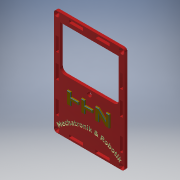
# Autodesk Inventor part: Deckplatte
Saved by Autodesk Inventor 2019 (Build 230136000, 136)
## iProperties
Created: 2022-10-31
Part Number: Deckplatte
Material: Generisch
Document SubType Name: Modeling
Designer: RP
Density: 1 g/cm^3
Appearance: Hellrot
Author: RP
Autodesk Inventor part; units mm, degrees
ref_plane "YZ Plane" through (0, 0, 0) normal (1, 0, 0) x (0, 1, 0)
ref_plane "XZ Plane" through (0, 0, 0) normal (0, 1, 0) x (-1, 0, 0)
sketch "Skizze1" plane through (0, 0, 0) normal (0, 0, 1) x (1, 0, 0)
  line L0 (92, 4) -> (0, 4)
  line L1 (96, -142) -> (96, 0)
  arc A0 (96, 0) -> (92, 4) centre (92, 0) ccw
  arc A1 (0, 4) -> (-4, 0) centre (0, 0) ccw
  line L2 (-4, 0) -> (-4, -142)
  arc A2 (-4, -142) -> (0, -146) centre (0, -142) ccw
  line L3 (0, -146) -> (92, -146)
  arc A3 (92, -146) -> (96, -142) centre (92, -142) ccw
  circle A4 centre (92, -142) radius 1.75
  circle A5 centre (0, -142) radius 1.75
  line L4 (37.25, -139.5) -> (17.25, -139.5)
  line L5 (17.25, -143.5) -> (37.25, -143.5)
  line L6 (17.25, -139.5) -> (17.25, -143.5)
  line L7 (37.25, -143.5) -> (37.25, -139.5)
  line L8 (54.75, -139.5) -> (54.75, -143.5)
  line L9 (74.75, -139.5) -> (54.75, -139.5)
  line L10 (54.75, -143.5) -> (74.75, -143.5)
  line L11 (74.75, -143.5) -> (74.75, -139.5)
  line L12 (89.5, -104.75) -> (89.5, -124.75)
  line L13 (93.5, -104.75) -> (89.5, -104.75)
  line L14 (93.5, -124.75) -> (93.5, -104.75)
  line L15 (89.5, -124.75) -> (93.5, -124.75)
  line L16 (93.5, -81) -> (93.5, -61)
  line L17 (89.5, -61) -> (89.5, -81)
  line L18 (89.5, -81) -> (93.5, -81)
  line L19 (93.5, -61) -> (89.5, -61)
  line L20 (89.5, -47) -> (93.5, -47)
  line L21 (93.5, -27) -> (89.5, -27)
  line L22 (93.5, -47) -> (93.5, -27)
  line L23 (89.5, -27) -> (89.5, -47)
  circle A6 centre (92, 0) radius 1.75
  line L24 (54.75, -2.5) -> (74.75, -2.5)
  line L25 (74.75, -2.5) -> (74.75, 1.5)
  line L26 (74.75, 1.5) -> (54.75, 1.5)
  line L27 (54.75, 1.5) -> (54.75, -2.5)
  line L28 (37.25, -2.5) -> (37.25, 1.5)
  line L29 (17.25, 1.5) -> (17.25, -2.5)
  line L30 (37.25, 1.5) -> (17.25, 1.5)
  line L31 (17.25, -2.5) -> (37.25, -2.5)
  circle A7 centre (0, 0) radius 1.75
  line L32 (2.5, -47) -> (2.5, -27)
  line L33 (-1.5, -27) -> (-1.5, -47)
  line L34 (2.5, -27) -> (-1.5, -27)
  line L35 (-1.5, -47) -> (2.5, -47)
  line L36 (2.5, -61) -> (-1.5, -61)
  line L37 (-1.5, -81) -> (2.5, -81)
  line L38 (2.5, -81) -> (2.5, -61)
  line L39 (-1.5, -61) -> (-1.5, -81)
  line L40 (-1.5, -104.75) -> (-1.5, -124.75)
  line L41 (2.5, -104.75) -> (-1.5, -104.75)
  line L42 (-1.5, -124.75) -> (2.5, -124.75)
  line L43 (2.5, -124.75) -> (2.5, -104.75)
  line L44 (4.4, -8) -> (87.6, -8)
  line L45 (87.6, -8) -> (87.6, -69.6)
  line L46 (87.6, -69.6) -> (4.4, -69.6)
  line L47 (4.4, -69.6) -> (4.4, -8)
  circle A8 centre (46, -76) radius 3.25
  line L48 (-4, -76) -> (96, -76) construction
  dimension "d0" = 8
  dimension "d1" = 4.4
  dimension "d2" = 4.4
  dimension "d3" = 69.6
  dimension "d7" = 6.5
  dimension "d8" = 76
  constraints: 98 end point, 23 horizontal, 22 vertical, 9 centre point, 8 point on circle, 2 parallel, 2 perpendicular, 2 point on line, 1 coincident, 1 midpoint, 64 other
  measures "d0" distance from line of L44 A0.centre
  measures "d1" distance from line of A0.centre L45
  measures "d2" distance from line of point (0, 0) L47
  measures "d3" distance from line of point (0, 0) L46
  measures "d7" diameter of A8
  measures "d8" vertical distance of point (0, 0) point (46, -76)
extrude "Extrusion1" add sketch "Skizze1" against normal blind 4
fillet "Rundung1" radius 6.6 2 edges at (4.4, -69.6, -2) (87.6, -69.6, -2)
chamfer "Fase2" distance 4 angle 45 1 edges at (46, -8, -4) measured on face at (46, -8, -3.5)
chamfer "Fase3" distance 2.2 angle 45 4 edges at (-1.75, -142, 0) (90.25, -142, 0) (-1.75, 0, 0) (90.25, 0, 0)
sketch "Skizze2" plane through (0, 0, 0) normal (0, 0, 1) x (1, 0, 0)
  line L0 (16, -85) -> (16, -102.0769)
  line L1 (16, -102.0769) -> (20.99, -102.0769)
  line L2 (20.99, -102.0769) -> (20.99, -95.5345)
  line L3 (20.99, -95.5345) -> (32.008, -95.5345)
  line L4 (32.008, -95.5345) -> (32.008, -91.5425)
  line L5 (32.008, -91.5425) -> (20.99, -91.5425)
  line L6 (20.99, -91.5425) -> (20.99, -85)
  line L7 (20.99, -85) -> (16, -85)
  line L8 (36, -85) -> (36, -102.0769)
  line L9 (36, -102.0769) -> (40.99, -102.0769)
  line L10 (40.99, -102.0769) -> (40.99, -95.5345)
  line L11 (40.99, -95.5345) -> (52.008, -95.5345)
  line L12 (52.008, -95.5345) -> (52.008, -91.5425)
  line L13 (52.008, -91.5425) -> (40.99, -91.5425)
  line L14 (40.99, -85) -> (40.99, -91.5425)
  line L15 (36, -85) -> (40.99, -85)
  line L16 (56, -85) -> (56, -102.0769)
  line L17 (56, -102.0769) -> (60.99, -102.0769)
  line L18 (71.01, -102.0769) -> (76, -102.0769)
  line L19 (76, -102.0769) -> (76, -85)
  line L20 (76, -85) -> (71.01, -85)
  line L21 (56, -85) -> (60.99, -85)
  circle A0 centre (92, 0) radius 1.75 construction
  circle A1 centre (92, -142) radius 1.75 construction
  circle A2 centre (0, -142) radius 1.75 construction
  line L22 (0, 0) -> (92, 0) construction
  line L23 (92, 0) -> (92, -142) construction
  line L24 (92, -142) -> (0, -142) construction
  line L25 (0, -142) -> (0, 0) construction
  line L26 (32.008, -93.5385) -> (16, -93.5385) construction
  line L27 (52.008, -93.5385) -> (36, -93.5385) construction
  line L28 (36, -93.5385) -> (32.008, -93.5385) construction
  line L29 (76, -93.5385) -> (56, -93.5385) construction
  line L30 (56, -93.5385) -> (52.008, -93.5385) construction
  line L31 (16, -85) -> (36, -85) construction
  line L32 (56, -85) -> (36, -85) construction
  line L33 (76, -85) -> (56, -85) construction
  line L34 (46, -76) -> (46, -60.5619) construction
  circle A3 centre (0, 0) radius 3.95 construction
  circle A4 centre (0, -142) radius 3.95 construction
  line L35 (4.4, -63) -> (4.4, -8) construction
  line L36 (87.6, -8) -> (87.6, -63) construction
  arc A5 (81, -69.6) -> (87.6, -63) centre (81, -63) ccw construction
  line L37 (81, -69.6) -> (11, -69.6) projected
  arc A6 (4.4, -63) -> (11, -69.6) centre (11, -63) ccw construction
  line L38 (2.5, -124.75) -> (-1.5, -124.75) construction
  line L39 (-1.5, -124.75) -> (-1.5, -104.75) construction
  line L40 (-1.5, -104.75) -> (2.5, -104.75) construction
  line L41 (2.5, -104.75) -> (2.5, -124.75) construction
  line L42 (-1.5, -81) -> (-1.5, -61) construction
  line L43 (-1.5, -61) -> (2.5, -61) construction
  line L44 (2.5, -61) -> (2.5, -81) construction
  line L45 (2.5, -81) -> (-1.5, -81) construction
  line L46 (-1.5, -27) -> (2.5, -27) construction
  line L47 (2.5, -27) -> (2.5, -47) construction
  line L48 (2.5, -47) -> (-1.5, -47) construction
  line L49 (-1.5, -47) -> (-1.5, -27) construction
  line L50 (17.25, 1.5) -> (37.25, 1.5) construction
  line L51 (37.25, 1.5) -> (37.25, -2.5) construction
  line L52 (37.25, -2.5) -> (17.25, -2.5) construction
  line L53 (17.25, -2.5) -> (17.25, 1.5) construction
  line L54 (74.75, 1.5) -> (74.75, -2.5) construction
  line L55 (74.75, -2.5) -> (54.75, -2.5) construction
  line L56 (54.75, -2.5) -> (54.75, 1.5) construction
  line L57 (54.75, 1.5) -> (74.75, 1.5) construction
  line L58 (93.5, -27) -> (93.5, -47) construction
  line L59 (93.5, -47) -> (89.5, -47) construction
  line L60 (89.5, -47) -> (89.5, -27) construction
  line L61 (89.5, -27) -> (93.5, -27) construction
  line L62 (89.5, -61) -> (93.5, -61) construction
  line L63 (93.5, -61) -> (93.5, -81) construction
  line L64 (93.5, -81) -> (89.5, -81) construction
  line L65 (89.5, -81) -> (89.5, -61) construction
  line L66 (93.5, -124.75) -> (89.5, -124.75) construction
  line L67 (89.5, -124.75) -> (89.5, -104.75) construction
  line L68 (89.5, -104.75) -> (93.5, -104.75) construction
  line L69 (93.5, -104.75) -> (93.5, -124.75) construction
  line L70 (74.75, -143.5) -> (54.75, -143.5) construction
  line L71 (54.75, -143.5) -> (54.75, -139.5) construction
  line L72 (54.75, -139.5) -> (74.75, -139.5) construction
  line L73 (74.75, -139.5) -> (74.75, -143.5) construction
  line L74 (17.25, -143.5) -> (17.25, -139.5) construction
  line L75 (17.25, -139.5) -> (37.25, -139.5) construction
  line L76 (37.25, -139.5) -> (37.25, -143.5) construction
  line L77 (37.25, -143.5) -> (17.25, -143.5) construction
  circle A7 centre (46, -76) radius 3.25 construction
  line L78 (92, 4) -> (0, 4) construction
  arc A8 (0, 4) -> (-4, 0) centre (0, 0) ccw construction
  line L79 (-4, 0) -> (-4, -142) construction
  arc A9 (-4, -142) -> (0, -146) centre (0, -142) ccw construction
  line L80 (0, -146) -> (92, -146) construction
  arc A10 (92, -146) -> (96, -142) centre (92, -142) ccw construction
  line L81 (96, -142) -> (96, 0) construction
  arc A11 (96, 0) -> (92, 4) centre (92, 0) ccw construction
  circle A12 centre (92, -142) radius 3.95 construction
  circle A13 centre (92, 0) radius 3.95 construction
  line L82 (71.01, -95.02) -> (60.99, -85)
  line L83 (71.01, -95.02) -> (71.01, -85)
  line L84 (60.99, -102.0769) -> (60.99, -92.0569)
  line L85 (60.99, -92.0569) -> (71.01, -102.0769)
  line L86 (73.2066, -97.2166) -> (69.6781, -100.7451) construction
  line L87 (4.4, -8) -> (87.6, -8) projected
  dimension "d19" = 60
  dimension "d20" = 45
  dimension "d22" = 3.992
  dimension "d23" = 4.99
  dimension "d24" = 17.0769
  dimension "d26" = 85
  dimension "d27" = 4.99
  constraints: 81 end point, 17 point on line, 16 perpendicular, 9 equal length, 6 midpoint, 5 collinear, 5 vertical, 3 horizontal, 3 parallel, 1 coincident, 1 other
  measures "d19" distance between parallel lines of L19 L0
  measures "d20" angle of L84 L85
  measures "d22" distance of L3.end L4.end
  measures "d23" distance between parallel lines of L2 L0
  measures "d24" distance between parallel lines of L1 L7
  measures "d26" distance from line of L7 L22.start
  measures "d27" distance between parallel lines of L82 L85
extrude "Extrusion2" add sketch "Skizze2" along normal blind 2
fillet "Rundung2" radius 0.5 25 edges at (26.499, -95.5345, 0) (20.99, -98.8057, 0) (18.495, -102.0769, 0) (32.008, -93.5385, 0) (40.99, -98.8057, 0) (46.499, -95.5345, 0) (38.495, -102.0769, 0) (58.495, -102.0769, 0) (60.99, -97.0669, 0) (66, -97.0669, 0) (73.505, -102.0769, 0) (76, -93.5385, 0) (73.505, -85, 0) (66, -90.01, 0) (58.495, -85, 0) (52.008, -93.5385, 0) (46.499, -91.5425, 0) (40.99, -88.2712, 0) (38.495, -85, 0) (26.499, -91.5425, 0) (20.99, -88.2712, 0) (18.495, -85, 0) (56, -93.5385, 0) (36, -93.5385, 0) (16, -93.5385, 0)
ref_plane "Arbeitsebene1" through (31.625, -139.5, 0) normal (0, -0.052336, 0.9986295) x (1, 0, 0)
sketch "Skizze3" plane through (31.625, -139.5, 0) normal (0, -0.052336, 0.9986295) x (1, 0, 0)
  arc A0 (52.375, 5.3883) -> (-23.625, 5.3883) centre (14.375, -43.5326) ccw construction
  ellipse E0 centre (14.375, 63.413) end of major axis (11.125, 63.413) minor radius 3.2455 construction
  line L0 (14.375, 63.413) -> (14.375, -10.3592) construction
  line L1 (14.375, -43.5326) -> (-23.625, 5.3883) construction
  line L2 (52.375, 5.3883) -> (14.375, -43.5326) construction
  ellipse E1 centre (-31.625, -2.6117) end of major axis (-33.375, -2.6117) minor radius 1.7476 construction
  line L3 (-35.625, 139.3088) -> (-35.625, -2.4966) construction
  line L4 (64.375, -2.4966) -> (64.375, 139.3088) construction
  line L5 (-23.8311, 5.3236) -> (-24.9638, 4.3439)
  line L6 (-24.9638, 4.3439) -> (-27.5657, 7.3521)
  line L7 (-27.5657, 7.3521) -> (-26.71, 4.6979)
  line L8 (-26.71, 4.6979) -> (-27.4896, 4.0236)
  line L9 (-27.4896, 4.0236) -> (-29.9928, 5.2529)
  line L10 (-29.9928, 5.2529) -> (-27.391, 2.2446)
  line L11 (-27.391, 2.2446) -> (-28.4648, 1.3159)
  line L12 (-28.4648, 1.3159) -> (-32.3899, 5.8539)
  line L13 (-32.3899, 5.8539) -> (-31.077, 6.9895)
  line L14 (-31.077, 6.9895) -> (-28.1323, 5.6214)
  line L15 (-28.1323, 5.6214) -> (-29.069, 8.7261)
  line L16 (-29.069, 8.7261) -> (-27.7562, 9.8617)
  line L17 (-27.7562, 9.8617) -> (-23.8311, 5.3236)
  spline S0 degree 2 poles (-20.9166, 7.2303) (-21.9657, 6.4907) (-23.7884, 6.7048) (-24.4412, 7.6307) knots 0 0 0 1 2 2 2
  spline S1 degree 2 poles (-24.4412, 7.6307) (-25.08, 8.5367) (-24.801, 10.3516) (-23.8632, 11.0129) knots 0 0 0 1 2 2 2
  spline S2 degree 2 poles (-23.8632, 11.0129) (-23.0168, 11.6097) (-21.5112, 11.2969) (-20.9116, 10.4465) knots 0 0 0 1 2 2 2
  line L18 (-20.9116, 10.4465) -> (-20.6174, 10.0293)
  line L19 (-20.6174, 10.0293) -> (-23.1487, 8.2445)
  spline S3 degree 2 poles (-23.1487, 8.2445) (-22.9507, 7.9974) (-22.523, 7.7873) (-22.2991, 7.7905) knots 0 0 0 1 2 2 2
  spline S4 degree 2 poles (-22.2991, 7.7905) (-22.0793, 7.7908) (-21.6202, 7.9836) (-21.3858, 8.1489) knots 0 0 0 1 2 2 2
  spline S5 degree 2 poles (-21.3858, 8.1489) (-21.1871, 8.289) (-20.8593, 8.651) (-20.7496, 8.8414) knots 0 0 0 1 2 2 2
  spline S6 degree 2 poles (-20.7496, 8.8414) (-20.6486, 9.0018) (-20.5138, 9.317) (-20.4775, 9.4259) knots 0 0 0 1 2 2 2
  line L20 (-20.4775, 9.4259) -> (-20.3544, 9.5127)
  line L21 (-20.3544, 9.5127) -> (-19.6819, 8.559)
  spline S7 degree 2 poles (-19.6819, 8.559) (-19.7857, 8.4025) (-19.949, 8.1446) (-20.122, 7.9512) knots 0 0 0 1 2 2 2
  spline S8 degree 2 poles (-20.122, 7.9512) (-20.2723, 7.7679) (-20.6305, 7.4321) (-20.9166, 7.2303) knots 0 0 0 1 2 2 2
  spline S9 degree 2 poles (-22.2442, 9.9233) (-22.51, 10.2833) (-23.1036, 10.4418) (-23.4334, 10.2093) knots 0 0 0 1 2 2 2
  spline S10 degree 2 poles (-23.4334, 10.2093) (-23.7712, 9.9711) (-23.8669, 9.2968) (-23.643, 8.9371) knots 0 0 0 1 2 2 2
  line L22 (-23.643, 8.9371) -> (-22.2442, 9.9233)
  spline S11 degree 2 poles (-16.8843, 9.8097) (-17.364, 9.5225) (-18.3057, 9.2874) (-18.7517, 9.3604) knots 0 0 0 1 2 2 2
  spline S12 degree 2 poles (-18.7517, 9.3604) (-19.1919, 9.4425) (-19.9744, 10.0111) (-20.2841, 10.5284) knots 0 0 0 1 2 2 2
  spline S13 degree 2 poles (-20.2841, 10.5284) (-20.6188, 11.0874) (-20.7354, 12.0773) (-20.5808, 12.51) knots 0 0 0 1 2 2 2
  spline S14 degree 2 poles (-20.5808, 12.51) (-20.4378, 12.9243) (-19.7934, 13.6274) (-19.3678, 13.8822) knots 0 0 0 1 2 2 2
  spline S15 degree 2 poles (-19.3678, 13.8822) (-19.0466, 14.0745) (-18.3143, 14.309) (-17.8915, 14.3411) knots 0 0 0 1 2 2 2
  line L23 (-17.8915, 14.3411) -> (-17.2721, 13.3065)
  line L24 (-17.2721, 13.3065) -> (-17.4264, 13.2141)
  spline S16 degree 2 poles (-17.4264, 13.2141) (-17.544, 13.24) (-17.8524, 13.282) (-18.0176, 13.2738) knots 0 0 0 1 2 2 2
  spline S17 degree 2 poles (-18.0176, 13.2738) (-18.196, 13.269) (-18.5855, 13.1718) (-18.7899, 13.0494) knots 0 0 0 1 2 2 2
  spline S18 degree 2 poles (-18.7899, 13.0494) (-19.253, 12.7722) (-19.3748, 11.8209) (-19.0451, 11.2702) knots 0 0 0 1 2 2 2
  spline S19 degree 2 poles (-19.0451, 11.2702) (-18.6955, 10.6862) (-17.8085, 10.4352) (-17.3579, 10.7049) knots 0 0 0 1 2 2 2
  spline S20 degree 2 poles (-17.3579, 10.7049) (-17.1285, 10.8423) (-16.8488, 11.1514) (-16.7686, 11.3014) knots 0 0 0 1 2 2 2
  spline S21 degree 2 poles (-16.7686, 11.3014) (-16.6901, 11.4447) (-16.6098, 11.7082) (-16.5847, 11.8082) knots 0 0 0 1 2 2 2
  line L25 (-16.5847, 11.8082) -> (-16.4303, 11.9006)
  line L26 (-16.4303, 11.9006) -> (-15.8084, 10.8619)
  spline S22 degree 2 poles (-15.8084, 10.8619) (-15.8853, 10.7535) (-16.0865, 10.4744) (-16.2058, 10.3519) knots 0 0 0 1 2 2 2
  spline S23 degree 2 poles (-16.2058, 10.3519) (-16.3511, 10.197) (-16.6298, 9.9621) (-16.8843, 9.8097) knots 0 0 0 1 2 2 2
  line L27 (-11.3125, 12.8763) -> (-12.5836, 12.2437)
  line L28 (-12.5836, 12.2437) -> (-13.5822, 14.2505)
  spline S24 degree 2 poles (-13.5822, 14.2505) (-13.7057, 14.4986) (-13.9875, 14.9666) (-14.096, 15.0538) knots 0 0 0 1 2 2 2
  spline S25 degree 2 poles (-14.096, 15.0538) (-14.2306, 15.1606) (-14.5329, 15.1569) (-14.7419, 15.0529) knots 0 0 0 1 2 2 2
  spline S26 degree 2 poles (-14.7419, 15.0529) (-14.8942, 14.9771) (-15.1535, 14.7014) (-15.2691, 14.4863) knots 0 0 0 1 2 2 2
  line L29 (-15.2691, 14.4863) -> (-13.8416, 11.6177)
  line L30 (-13.8416, 11.6177) -> (-15.1039, 10.9895)
  line L31 (-15.1039, 10.9895) -> (-17.8963, 16.6005)
  line L32 (-17.8963, 16.6005) -> (-16.6339, 17.2287)
  line L33 (-16.6339, 17.2287) -> (-15.6352, 15.222)
  spline S27 degree 2 poles (-15.6352, 15.222) (-15.4561, 15.637) (-15.0158, 16.2254) (-14.6589, 16.4031) knots 0 0 0 1 2 2 2
  spline S28 degree 2 poles (-14.6589, 16.4031) (-14.0407, 16.7107) (-12.9935, 16.2542) (-12.6252, 15.5142) knots 0 0 0 1 2 2 2
  line L34 (-12.6252, 15.5142) -> (-11.3125, 12.8763)
  spline S29 degree 2 poles (-8.2168, 14.6658) (-8.3073, 14.4989) (-8.4475, 14.2336) (-8.5922, 14.0712) knots 0 0 0 1 2 2 2
  spline S30 degree 2 poles (-8.5922, 14.0712) (-8.7341, 13.9152) (-9.0323, 13.6916) (-9.3304, 13.5728) knots 0 0 0 1 2 2 2
  spline S31 degree 2 poles (-9.3304, 13.5728) (-9.8905, 13.3495) (-10.9256, 13.8058) (-11.1524, 14.3749) knots 0 0 0 1 2 2 2
  spline S32 degree 2 poles (-11.1524, 14.3749) (-11.3379, 14.8401) (-11.1935, 15.5677) (-10.9078, 15.8753) knots 0 0 0 1 2 2 2
  spline S33 degree 2 poles (-10.9078, 15.8753) (-10.6194, 16.1891) (-9.6842, 16.7189) (-9.1296, 16.9819) knots 0 0 0 1 2 2 2
  line L35 (-9.1296, 16.9819) -> (-9.1386, 17.0045)
  spline S34 degree 2 poles (-9.1386, 17.0045) (-9.2772, 17.3523) (-9.8983, 17.4135) (-10.4132, 17.2082) knots 0 0 0 1 2 2 2
  spline S35 degree 2 poles (-10.4132, 17.2082) (-10.6435, 17.1164) (-11.2002, 16.7009) (-11.4416, 16.4528) knots 0 0 0 1 2 2 2
  line L36 (-11.4416, 16.4528) -> (-11.5545, 16.4078)
  line L37 (-11.5545, 16.4078) -> (-11.9596, 17.4241)
  spline S36 degree 2 poles (-11.9596, 17.4241) (-11.787, 17.5557) (-10.981, 18.0549) (-10.5384, 18.2314) knots 0 0 0 1 2 2 2
  spline S37 degree 2 poles (-10.5384, 18.2314) (-9.4544, 18.6635) (-8.1727, 18.3369) (-7.8774, 17.5962) knots 0 0 0 1 2 2 2
  line L38 (-7.8774, 17.5962) -> (-6.7377, 14.7372)
  line L39 (-6.7377, 14.7372) -> (-8.0385, 14.2186)
  line L40 (-8.0385, 14.2186) -> (-8.2168, 14.6658)
  line L41 (-8.476, 15.3162) -> (-8.8235, 16.1879)
  spline S38 degree 2 poles (-8.8235, 16.1879) (-9.1451, 16.023) (-9.5364, 15.8095) (-9.7063, 15.658) knots 0 0 0 1 2 2 2
  spline S39 degree 2 poles (-9.7063, 15.658) (-9.859, 15.5291) (-9.9515, 15.2096) (-9.8723, 15.0109) knots 0 0 0 1 2 2 2
  spline S40 degree 2 poles (-9.8723, 15.0109) (-9.7552, 14.7173) (-9.3463, 14.6238) (-9.0347, 14.748) knots 0 0 0 1 2 2 2
  spline S41 degree 2 poles (-9.0347, 14.748) (-8.8631, 14.8164) (-8.5648, 15.1185) (-8.476, 15.3162) knots 0 0 0 1 2 2 2
  spline S42 degree 2 poles (-4.0715, 15.5136) (-4.8906, 15.2496) (-5.8581, 15.6836) (-6.1057, 16.4518) knots 0 0 0 1 2 2 2
  line L42 (-6.1057, 16.4518) -> (-6.7545, 18.4649)
  line L43 (-6.7545, 18.4649) -> (-7.2682, 18.2994)
  line L44 (-7.2682, 18.2994) -> (-7.5695, 19.2342)
  line L45 (-7.5695, 19.2342) -> (-7.0558, 19.3997)
  line L46 (-7.0558, 19.3997) -> (-7.4526, 20.6307)
  line L47 (-7.4526, 20.6307) -> (-6.1106, 21.0633)
  line L48 (-6.1106, 21.0633) -> (-5.7138, 19.8323)
  line L49 (-5.7138, 19.8323) -> (-4.418, 20.25)
  line L50 (-4.418, 20.25) -> (-4.1167, 19.3151)
  line L51 (-4.1167, 19.3151) -> (-5.4125, 18.8975)
  line L52 (-5.4125, 18.8975) -> (-4.9188, 17.3657)
  spline S43 degree 2 poles (-4.9188, 17.3657) (-4.8457, 17.1389) (-4.7275, 16.8041) (-4.6287, 16.6878) knots 0 0 0 1 2 2 2
  spline S44 degree 2 poles (-4.6287, 16.6878) (-4.53, 16.5715) (-4.2062, 16.5021) (-3.947, 16.5857) knots 0 0 0 1 2 2 2
  spline S45 degree 2 poles (-3.947, 16.5857) (-3.836, 16.6215) (-3.5187, 16.8259) (-3.4612, 16.8853) knots 0 0 0 1 2 2 2
  line L53 (-3.4612, 16.8853) -> (-3.3455, 16.9226)
  line L54 (-3.3455, 16.9226) -> (-3.0413, 15.9785)
  spline S46 degree 2 poles (-3.0413, 15.9785) (-3.2409, 15.8529) (-3.7105, 15.63) (-4.0715, 15.5136) knots 0 0 0 1 2 2 2
  line L55 (-0.3403, 19.9438) -> (-0.4532, 19.9144)
  spline S47 degree 2 poles (-0.4532, 19.9144) (-0.5405, 19.9217) (-0.8443, 19.8726) (-1.0231, 19.826) knots 0 0 0 1 2 2 2
  spline S48 degree 2 poles (-1.0231, 19.826) (-1.2348, 19.7707) (-1.6768, 19.5197) (-1.8758, 19.3773) knots 0 0 0 1 2 2 2
  line L56 (-1.8758, 19.3773) -> (-1.1109, 16.4463)
  line L57 (-1.1109, 16.4463) -> (-2.4753, 16.0902)
  line L58 (-2.4753, 16.0902) -> (-3.6183, 20.4703)
  line L59 (-3.6183, 20.4703) -> (-2.2539, 20.8263)
  line L60 (-2.2539, 20.8263) -> (-2.0894, 20.1959)
  spline S49 degree 2 poles (-2.0894, 20.1959) (-2.0174, 20.3051) (-1.7569, 20.6545) (-1.6413, 20.7701) knots 0 0 0 1 2 2 2
  spline S50 degree 2 poles (-1.6413, 20.7701) (-1.5141, 20.8988) (-1.152, 21.129) (-0.978, 21.1744) knots 0 0 0 1 2 2 2
  spline S51 degree 2 poles (-0.978, 21.1744) (-0.9121, 21.1916) (-0.745, 21.2251) (-0.6779, 21.2376) knots 0 0 0 1 2 2 2
  line L61 (-0.6779, 21.2376) -> (-0.3403, 19.9438)
  spline S52 degree 2 poles (4.8407, 20.005) (5.0467, 18.9059) (4.0837, 17.4193) (2.9894, 17.2142) knots 0 0 0 1 2 2 2
  spline S53 degree 2 poles (2.9894, 17.2142) (1.8997, 17.0099) (0.4541, 18.0449) (0.2481, 19.1441) knots 0 0 0 1 2 2 2
  spline S54 degree 2 poles (0.2481, 19.1441) (0.0402, 20.2528) (1.0137, 21.7363) (2.1033, 21.9406) knots 0 0 0 1 2 2 2
  spline S55 degree 2 poles (2.1033, 21.9406) (3.1929, 22.1449) (4.6337, 21.109) (4.8407, 20.005) knots 0 0 0 1 2 2 2
  spline S56 degree 2 poles (3.4231, 19.7294) (3.3488, 20.1261) (3.1203, 20.6323) (2.976, 20.7685) knots 0 0 0 1 2 2 2
  spline S57 degree 2 poles (2.976, 20.7685) (2.8204, 20.9125) (2.4856, 20.9833) (2.2897, 20.9466) knots 0 0 0 1 2 2 2
  spline S58 degree 2 poles (2.2897, 20.9466) (2.0985, 20.9107) (1.8189, 20.7396) (1.7251, 20.5538) knots 0 0 0 1 2 2 2
  spline S59 degree 2 poles (1.7251, 20.5538) (1.6343, 20.3785) (1.5922, 19.8116) (1.6692, 19.4006) knots 0 0 0 1 2 2 2
  spline S60 degree 2 poles (1.6692, 19.4006) (1.7454, 18.9944) (1.9733, 18.5177) (2.1119, 18.3854) knots 0 0 0 1 2 2 2
  spline S61 degree 2 poles (2.1119, 18.3854) (2.2504, 18.253) (2.6118, 18.1724) (2.8126, 18.21) knots 0 0 0 1 2 2 2
  spline S62 degree 2 poles (2.8126, 18.21) (2.9798, 18.2414) (3.297, 18.4492) (3.3753, 18.6123) knots 0 0 0 1 2 2 2
  spline S63 degree 2 poles (3.3753, 18.6123) (3.4634, 18.802) (3.502, 19.3088) (3.4231, 19.7294) knots 0 0 0 1 2 2 2
  line L62 (10.2123, 18.3098) -> (8.7998, 18.1657)
  line L63 (8.7998, 18.1657) -> (8.5724, 20.3956)
  spline S64 degree 2 poles (8.5724, 20.3956) (8.5442, 20.6714) (8.4455, 21.2087) (8.3746, 21.3285) knots 0 0 0 1 2 2 2
  spline S65 degree 2 poles (8.3746, 21.3285) (8.2862, 21.4759) (8.002, 21.5789) (7.7698, 21.5552) knots 0 0 0 1 2 2 2
  spline S66 degree 2 poles (7.7698, 21.5552) (7.6005, 21.5379) (7.2608, 21.3713) (7.0767, 21.2108) knots 0 0 0 1 2 2 2
  line L64 (7.0767, 21.2108) -> (7.4019, 18.0231)
  line L65 (7.4019, 18.0231) -> (5.9991, 17.88)
  line L66 (5.9991, 17.88) -> (5.5398, 22.3834)
  line L67 (5.5398, 22.3834) -> (6.9425, 22.5265)
  line L68 (6.9425, 22.5265) -> (6.9934, 22.0283)
  spline S67 degree 2 poles (6.9934, 22.0283) (7.3072, 22.3535) (7.9266, 22.7491) (8.3233, 22.7895) knots 0 0 0 1 2 2 2
  spline S68 degree 2 poles (8.3233, 22.7895) (9.0102, 22.8596) (9.8294, 22.0634) (9.9133, 21.2411) knots 0 0 0 1 2 2 2
  line L69 (9.9133, 21.2411) -> (10.2123, 18.3098)
  line L70 (12.6662, 18.3934) -> (11.2572, 18.3385)
  line L71 (11.2572, 18.3385) -> (11.0809, 22.8618)
  line L72 (11.0809, 22.8618) -> (12.4898, 22.9167)
  line L73 (12.4898, 22.9167) -> (12.6662, 18.3934)
  line L74 (12.5084, 23.5646) -> (11.0168, 23.5065)
  line L75 (11.0168, 23.5065) -> (10.974, 24.6045)
  line L76 (10.974, 24.6045) -> (12.4656, 24.6626)
  line L77 (12.4656, 24.6626) -> (12.5084, 23.5646)
  line L78 (18.275, 18.3441) -> (16.5979, 18.3797)
  line L79 (16.5979, 18.3797) -> (15.4146, 20.3697)
  line L80 (15.4146, 20.3697) -> (15.1897, 20.0826)
  line L81 (15.1897, 20.0826) -> (15.1541, 18.4104)
  line L82 (15.1541, 18.4104) -> (13.7444, 18.4404)
  line L83 (13.7444, 18.4404) -> (13.8776, 24.7064)
  line L84 (13.8776, 24.7064) -> (15.2873, 24.6764)
  line L85 (15.2873, 24.6764) -> (15.2127, 21.1667)
  line L86 (15.2127, 21.1667) -> (16.5871, 22.9077)
  line L87 (16.5871, 22.9077) -> (18.2545, 22.8723)
  line L88 (18.2545, 22.8723) -> (16.6283, 20.9566)
  line L89 (16.6283, 20.9566) -> (18.275, 18.3441)
  line L90 (27.1946, 17.1705) -> (25.4212, 17.4428)
  line L91 (25.4212, 17.4428) -> (24.9789, 18.0223)
  spline S69 degree 2 poles (24.9789, 18.0223) (24.5091, 17.7501) (23.5902, 17.5961) (23.1096, 17.6699) knots 0 0 0 1 2 2 2
  spline S70 degree 2 poles (23.1096, 17.6699) (22.0859, 17.8271) (21.0642, 19.022) (21.1897, 19.839) knots 0 0 0 1 2 2 2
  spline S71 degree 2 poles (21.1897, 19.839) (21.2435, 20.1898) (21.5063, 20.6512) (21.6862, 20.8302) knots 0 0 0 1 2 2 2
  spline S72 degree 2 poles (21.6862, 20.8302) (21.8544, 20.9962) (22.2776, 21.2215) (22.4757, 21.2943) knots 0 0 0 1 2 2 2
  spline S73 degree 2 poles (22.4757, 21.2943) (22.3241, 21.4603) (22.0941, 21.7563) (22.0183, 21.9352) knots 0 0 0 1 2 2 2
  spline S74 degree 2 poles (22.0183, 21.9352) (21.9362, 22.1052) (21.881, 22.4827) (21.9186, 22.7278) knots 0 0 0 1 2 2 2
  spline S75 degree 2 poles (21.9186, 22.7278) (21.9585, 22.9873) (22.2411, 23.4505) (22.5139, 23.6251) knots 0 0 0 1 2 2 2
  spline S76 degree 2 poles (22.5139, 23.6251) (22.7645, 23.7834) (23.6021, 23.9204) (24.1308, 23.8392) knots 0 0 0 1 2 2 2
  spline S77 degree 2 poles (24.1308, 23.8392) (24.6066, 23.7662) (25.2683, 23.4628) (25.478, 23.2585) knots 0 0 0 1 2 2 2
  spline S78 degree 2 poles (25.478, 23.2585) (25.6781, 23.0556) (25.8501, 22.5421) (25.808, 22.2682) knots 0 0 0 1 2 2 2
  spline S79 degree 2 poles (25.808, 22.2682) (25.7815, 22.0952) (25.6071, 21.6645) (25.4493, 21.5018) knots 0 0 0 1 2 2 2
  spline S80 degree 2 poles (25.4493, 21.5018) (25.2623, 21.3091) (24.7093, 21.0399) (24.3049, 20.9692) knots 0 0 0 1 2 2 2
  line L92 (24.3049, 20.9692) -> (25.2749, 19.6937)
  line L93 (25.2749, 19.6937) -> (25.4768, 20.9761)
  line L94 (25.4768, 20.9761) -> (26.8657, 20.7628)
  line L95 (26.8657, 20.7628) -> (26.7978, 20.3207)
  spline S81 degree 2 poles (26.7978, 20.3207) (26.7727, 20.1573) (26.6316, 19.687) (26.5474, 19.5229) knots 0 0 0 1 2 2 2
  spline S82 degree 2 poles (26.5474, 19.5229) (26.4602, 19.3395) (26.1852, 18.9587) (25.9931, 18.7963) knots 0 0 0 1 2 2 2
  line L96 (25.9931, 18.7963) -> (27.2071, 17.2522)
  line L97 (27.2071, 17.2522) -> (27.1946, 17.1705)
  line L98 (24.4294, 18.8003) -> (23.0655, 20.5544)
  spline S83 degree 2 poles (23.0655, 20.5544) (22.989, 20.4727) (22.7655, 20.0741) (22.7301, 19.8435) knots 0 0 0 1 2 2 2
  spline S84 degree 2 poles (22.7301, 19.8435) (22.6895, 19.5791) (22.8083, 19.1673) (22.9325, 19.0154) knots 0 0 0 1 2 2 2
  spline S85 degree 2 poles (22.9325, 19.0154) (23.0575, 18.8684) (23.3932, 18.684) (23.571, 18.6567) knots 0 0 0 1 2 2 2
  spline S86 degree 2 poles (23.571, 18.6567) (23.8209, 18.6183) (24.2183, 18.6753) (24.4294, 18.8003) knots 0 0 0 1 2 2 2
  spline S87 degree 2 poles (24.3486, 22.3103) (24.3796, 22.5122) (24.3115, 22.7735) (24.2353, 22.8541) knots 0 0 0 1 2 2 2
  spline S88 degree 2 poles (24.2353, 22.8541) (24.168, 22.9284) (23.9905, 22.99) (23.9377, 22.9982) knots 0 0 0 1 2 2 2
  spline S89 degree 2 poles (23.9377, 22.9982) (23.88, 23.007) (23.7307, 22.9955) (23.6242, 22.943) knots 0 0 0 1 2 2 2
  spline S90 degree 2 poles (23.6242, 22.943) (23.5447, 22.906) (23.3973, 22.6827) (23.3722, 22.5193) knots 0 0 0 1 2 2 2
  spline S91 degree 2 poles (23.3722, 22.5193) (23.336, 22.2838) (23.5905, 21.8266) (23.8338, 21.5531) knots 0 0 0 1 2 2 2
  spline S92 degree 2 poles (23.8338, 21.5531) (24.0526, 21.6966) (24.3109, 22.0652) (24.3486, 22.3103) knots 0 0 0 1 2 2 2
  line L99 (35.225, 14.8847) -> (33.4693, 15.4118)
  line L100 (33.4693, 15.4118) -> (32.5054, 18.001)
  line L101 (32.5054, 18.001) -> (31.9839, 18.1576)
  line L102 (31.9839, 18.1576) -> (31.3505, 16.048)
  line L103 (31.3505, 16.048) -> (29.9162, 16.4787)
  line L104 (29.9162, 16.4787) -> (31.6416, 22.2253)
  line L105 (31.6416, 22.2253) -> (33.9514, 21.5317)
  spline S93 degree 2 poles (33.9514, 21.5317) (34.431, 21.3877) (35.1025, 21.0541) (35.3493, 20.7769) knots 0 0 0 1 2 2 2
  spline S94 degree 2 poles (35.3493, 20.7769) (35.5979, 20.4891) (35.778, 19.77) (35.6382, 19.3043) knots 0 0 0 1 2 2 2
  spline S95 degree 2 poles (35.6382, 19.3043) (35.441, 18.6477) (34.5974, 18.0024) (34.0265, 17.9098) knots 0 0 0 1 2 2 2
  line L106 (34.0265, 17.9098) -> (35.225, 14.8847)
  spline S96 degree 2 poles (34.1027, 19.5673) (34.1685, 19.7862) (34.0945, 20.1485) (33.9287, 20.2897) knots 0 0 0 1 2 2 2
  spline S97 degree 2 poles (33.9287, 20.2897) (33.8105, 20.3861) (33.4896, 20.518) (33.2428, 20.5921) knots 0 0 0 1 2 2 2
  line L107 (33.2428, 20.5921) -> (32.7585, 20.7375)
  line L108 (32.7585, 20.7375) -> (32.2943, 19.1914)
  line L109 (32.2943, 19.1914) -> (32.7087, 19.067)
  spline S98 degree 2 poles (32.7087, 19.067) (33.0068, 18.9775) (33.4529, 18.9248) (33.6322, 18.9978) knots 0 0 0 1 2 2 2
  spline S99 degree 2 poles (33.6322, 18.9978) (33.8055, 19.0677) (34.03, 19.3251) (34.1027, 19.5673) knots 0 0 0 1 2 2 2
  spline S100 degree 2 poles (40.423, 15.1993) (40.0071, 14.1612) (38.3968, 13.4235) (37.3632, 13.8377) knots 0 0 0 1 2 2 2
  spline S101 degree 2 poles (37.3632, 13.8377) (36.3342, 14.25) (35.6697, 15.899) (36.0856, 16.9371) knots 0 0 0 1 2 2 2
  spline S102 degree 2 poles (36.0856, 16.9371) (36.5051, 17.9842) (38.1226, 18.7138) (39.1517, 18.3015) knots 0 0 0 1 2 2 2
  spline S103 degree 2 poles (39.1517, 18.3015) (40.1807, 17.8892) (40.8407, 16.2419) (40.423, 15.1993) knots 0 0 0 1 2 2 2
  spline S104 degree 2 poles (39.0789, 15.7273) (39.229, 16.102) (39.3078, 16.6518) (39.2592, 16.8441) knots 0 0 0 1 2 2 2
  spline S105 degree 2 poles (39.2592, 16.8441) (39.2051, 17.0491) (38.9606, 17.2885) (38.7755, 17.3627) knots 0 0 0 1 2 2 2
  spline S106 degree 2 poles (38.7755, 17.3627) (38.595, 17.435) (38.2673, 17.4406) (38.0884, 17.3342) knots 0 0 0 1 2 2 2
  spline S107 degree 2 poles (38.0884, 17.3342) (37.9177, 17.2349) (37.578, 16.7792) (37.4225, 16.391) knots 0 0 0 1 2 2 2
  spline S108 degree 2 poles (37.4225, 16.391) (37.2687, 16.0074) (37.2053, 15.4828) (37.2512, 15.2968) knots 0 0 0 1 2 2 2
  spline S109 degree 2 poles (37.2512, 15.2968) (37.2971, 15.1108) (37.5588, 14.8488) (37.7484, 14.7728) knots 0 0 0 1 2 2 2
  spline S110 degree 2 poles (37.7484, 14.7728) (37.9064, 14.7095) (38.2856, 14.7147) (38.4391, 14.8104) knots 0 0 0 1 2 2 2
  spline S111 degree 2 poles (38.4391, 14.8104) (38.6153, 14.9231) (38.9198, 15.3302) (39.0789, 15.7273) knots 0 0 0 1 2 2 2
  spline S112 degree 2 poles (45.2655, 12.8764) (44.7823, 11.9112) (43.2076, 11.2097) (42.4815, 11.5733) knots 0 0 0 1 2 2 2
  spline S113 degree 2 poles (42.4815, 11.5733) (42.1815, 11.7235) (41.8012, 12.0825) (41.6208, 12.3522) knots 0 0 0 1 2 2 2
  line L110 (41.6208, 12.3522) -> (41.4685, 12.1783)
  line L111 (41.4685, 12.1783) -> (40.2598, 12.7835)
  line L112 (40.2598, 12.7835) -> (43.0657, 18.3877)
  line L113 (43.0657, 18.3877) -> (44.3266, 17.7564)
  line L114 (44.3266, 17.7564) -> (43.334, 15.7739)
  spline S114 degree 2 poles (43.334, 15.7739) (43.7319, 15.8737) (44.4539, 15.882) (44.8321, 15.6926) knots 0 0 0 1 2 2 2
  spline S115 degree 2 poles (44.8321, 15.6926) (45.5408, 15.3378) (45.7553, 13.8547) (45.2655, 12.8764) knots 0 0 0 1 2 2 2
  spline S116 degree 2 poles (43.9612, 13.4969) (44.2637, 14.1012) (44.1576, 14.8014) (43.775, 14.993) knots 0 0 0 1 2 2 2
  spline S117 degree 2 poles (43.775, 14.993) (43.6054, 15.0779) (43.2162, 15.1368) (43.0009, 15.1087) knots 0 0 0 1 2 2 2
  line L115 (43.0009, 15.1087) -> (41.9865, 13.0826)
  spline S118 degree 2 poles (41.9865, 13.0826) (42.0865, 12.9673) (42.3256, 12.8041) (42.4517, 12.741) knots 0 0 0 1 2 2 2
  spline S119 degree 2 poles (42.4517, 12.741) (42.9082, 12.5124) (43.6586, 12.8925) (43.9612, 13.4969) knots 0 0 0 1 2 2 2
  spline S120 degree 2 poles (49.782, 10.0797) (49.2, 9.1247) (47.4899, 8.6637) (46.5391, 9.2431) knots 0 0 0 1 2 2 2
  spline S121 degree 2 poles (46.5391, 9.2431) (45.5924, 9.82) (45.2099, 11.5563) (45.7919, 12.5112) knots 0 0 0 1 2 2 2
  spline S122 degree 2 poles (45.7919, 12.5112) (46.3789, 13.4745) (48.0948, 13.9264) (49.0415, 13.3495) knots 0 0 0 1 2 2 2
  spline S123 degree 2 poles (49.0415, 13.3495) (49.9881, 12.7726) (50.3665, 11.0388) (49.782, 10.0797) knots 0 0 0 1 2 2 2
  spline S124 degree 2 poles (48.5438, 10.8229) (48.7538, 11.1675) (48.9225, 11.6967) (48.9064, 11.8944) knots 0 0 0 1 2 2 2
  spline S125 degree 2 poles (48.9064, 11.8944) (48.887, 12.1055) (48.6854, 12.3821) (48.5152, 12.4858) knots 0 0 0 1 2 2 2
  spline S126 degree 2 poles (48.5152, 12.4858) (48.3491, 12.587) (48.0268, 12.6468) (47.8328, 12.5714) knots 0 0 0 1 2 2 2
  spline S127 degree 2 poles (47.8328, 12.5714) (47.6481, 12.5018) (47.2376, 12.1085) (47.02, 11.7515) knots 0 0 0 1 2 2 2
  spline S128 degree 2 poles (47.02, 11.7515) (46.8049, 11.3985) (46.6555, 10.8917) (46.67, 10.7007) knots 0 0 0 1 2 2 2
  spline S129 degree 2 poles (46.67, 10.7007) (46.6846, 10.5096) (46.8993, 10.2079) (47.0737, 10.1017) knots 0 0 0 1 2 2 2
  spline S130 degree 2 poles (47.0737, 10.1017) (47.219, 10.0131) (47.5939, 9.9555) (47.7611, 10.0244) knots 0 0 0 1 2 2 2
  spline S131 degree 2 poles (47.7611, 10.0244) (47.9535, 10.1065) (48.3211, 10.4575) (48.5438, 10.8229) knots 0 0 0 1 2 2 2
  spline S132 degree 2 poles (50.5708, 6.633) (49.8684, 7.1303) (49.6357, 8.1648) (50.102, 8.8236) knots 0 0 0 1 2 2 2
  line L116 (50.102, 8.8236) -> (51.3241, 10.5498)
  line L117 (51.3241, 10.5498) -> (50.8836, 10.8617)
  line L118 (50.8836, 10.8617) -> (51.4511, 11.6633)
  line L119 (51.4511, 11.6633) -> (51.8916, 11.3515)
  line L120 (51.8916, 11.3515) -> (52.6389, 12.4071)
  line L121 (52.6389, 12.4071) -> (53.7898, 11.5924)
  line L122 (53.7898, 11.5924) -> (53.0425, 10.5368)
  line L123 (53.0425, 10.5368) -> (54.1537, 9.7501)
  line L124 (54.1537, 9.7501) -> (53.5862, 8.9485)
  line L125 (53.5862, 8.9485) -> (52.475, 9.7351)
  line L126 (52.475, 9.7351) -> (51.5451, 8.4216)
  spline S133 degree 2 poles (51.5451, 8.4216) (51.4074, 8.2271) (51.2103, 7.9318) (51.1764, 7.783) knots 0 0 0 1 2 2 2
  spline S134 degree 2 poles (51.1764, 7.783) (51.1426, 7.6342) (51.2812, 7.3335) (51.5034, 7.1762) knots 0 0 0 1 2 2 2
  spline S135 degree 2 poles (51.5034, 7.1762) (51.5987, 7.1088) (51.9525, 6.9774) (52.0345, 6.967) knots 0 0 0 1 2 2 2
  line L127 (52.0345, 6.967) -> (52.1337, 6.8968)
  line L128 (52.1337, 6.8968) -> (51.5606, 6.0872)
  spline S136 degree 2 poles (51.5606, 6.0872) (51.3404, 6.1717) (50.8804, 6.4139) (50.5708, 6.633) knots 0 0 0 1 2 2 2
  line L129 (53.0949, 4.8256) -> (51.9843, 5.6943)
  line L130 (51.9843, 5.6943) -> (54.7732, 9.2599)
  line L131 (54.7732, 9.2599) -> (55.8839, 8.3912)
  line L132 (55.8839, 8.3912) -> (53.0949, 4.8256)
  line L133 (56.3167, 8.8736) -> (55.141, 9.7933)
  line L134 (55.141, 9.7933) -> (55.818, 10.6588)
  line L135 (55.818, 10.6588) -> (56.9937, 9.7391)
  line L136 (56.9937, 9.7391) -> (56.3167, 8.8736)
  line L137 (57.3429, 1.1629) -> (56.0862, 2.2741)
  line L138 (56.0862, 2.2741) -> (56.4694, 4.5573)
  line L139 (56.4694, 4.5573) -> (56.1123, 4.4837)
  line L140 (56.1123, 4.4837) -> (55.0044, 3.2306)
  line L141 (55.0044, 3.2306) -> (53.948, 4.1646)
  line L142 (53.948, 4.1646) -> (58.0995, 8.8599)
  line L143 (58.0995, 8.8599) -> (59.1558, 7.9259)
  line L144 (59.1558, 7.9259) -> (56.8305, 5.296)
  line L145 (56.8305, 5.296) -> (59.0045, 5.7362)
  line L146 (59.0045, 5.7362) -> (60.2539, 4.6315)
  line L147 (60.2539, 4.6315) -> (57.775, 4.2207)
  line L148 (57.775, 4.2207) -> (57.3429, 1.1629)
  point P0 (-31.625, 139.3088)
  point P1 (14.375, 18.413)
  dimension "d32" = 45
  dimension "d33" = 8
  dimension "d34" = 8
  dimension "d35" = 75.678
  constraints: 6 end point, 3 point on circle, 2 point on line, 1 centre point, 1 vertical, 4 other
  measures "d32" distance of point (14.375, 18.413) L0.start
  measures "d33" horizontal distance of L1.end point (-31.625, -2.612)
  measures "d34" horizontal distance of point (-31.625, -2.612) L1.end
  measures "d35" angle of L2 L1
emboss "Prägen1" sketch "Skizze3" operation cut depth 1.5 direction (0, 0.052336, -0.9986295)
chamfer "Fase4" distance 0.5 angle 45 26 edges at (26.499, -91.5425, 2) (20.99, -88.2712, 2) (18.495, -85, 2) (16, -93.5385, 2) (18.495, -102.0769, 2) (20.99, -98.8057, 2) (26.499, -95.5345, 2) (32.008, -93.5385, 2) (36, -93.5385, 2) (38.495, -85, 2) (40.99, -88.2712, 2) (38.495, -102.0769, 2) (40.99, -98.8057, 2) (46.499, -95.5345, 2) (46.499, -91.5425, 2) (52.008, -93.5385, 2) (56, -93.5385, 2) (58.495, -102.0769, 2) (58.495, -85, 2) (66, -90.01, 2) (66, -97.0669, 2) (60.99, -97.0669, 2) (73.505, -102.0769, 2) (71.01, -90.01, 2) (76, -93.5385, 2) (73.505, -85, 2)
equation "\"d22\" = 0.8 * d23"
equation "\"d24\" = 0.284615 * d19"
equation "\"d27\" = d23"
